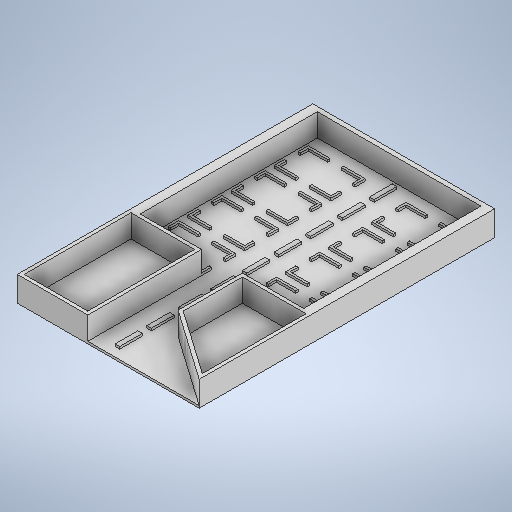
# Autodesk Inventor part: SchitaMacheta
Saved by Autodesk Inventor 2025 (Build 290162010, 162A)
## iProperties
Created: 2026-06-09
Part Number: SchitaMacheta
Material: Generic
Document SubType Name: Modeling
Designer: milot
Density: 1 g/cm^3
Appearance: Default
Author: milot
Autodesk Inventor part; units mm, degrees
ref_plane "YZ Plane" through (0, 0, 0) normal (1, 0, 0) x (0, 1, 0)
ref_plane "XZ Plane" through (0, 0, 0) normal (0, 1, 0) x (-1, 0, 0)
ref_plane "XY Plane" through (0, 0, 0) normal (0, 0, 1) x (1, 0, 0)
sketch "Sketch1" plane through (0, 0, 0) normal (0, 1, 0) x (-1, 0, 0)
  line L0 (-40, 65) -> (40, 65)
  line L1 (40, 65) -> (40, -65)
  line L2 (40, -65) -> (-40, -65)
  line L3 (-40, -65) -> (-40, 65)
  line L4 (-40, 65) -> (40, -65) construction
  line L5 (40, 65) -> (-40, -65) construction
  point P0 (0, 0)
  dimension "d0" = 130
  dimension "d1" = 80
  constraints: 12 end point, 2 midpoint, 2 parallel, 1 horizontal, 1 perpendicular
  measures "d0" distance of L0.end L1.end
  measures "d1" distance of L1.end L2.end
extrude "Extrusion1" add sketch "Sketch1" along normal blind 1
sketch "Sketch2" plane through (0, 1, 0) normal (0, 1, 0) x (1, 0, 0)
  line L0 (-40, -65) -> (40, -65) construction
  line L1 (0, -65) -> (-9, -65) construction
  line L2 (0, -65) -> (9, -65) construction
  line L3 (-9, -65) -> (9, -65)
  line L4 (9, -65) -> (9, 65)
  line L5 (-9, 85) -> (-9, -65)
  line L6 (1, -51) -> (-1, -51)
  line L7 (-1, -51) -> (-1, -61)
  line L8 (-1, -61) -> (1, -61)
  line L9 (1, -61) -> (1, -51)
  line L10 (1, -51) -> (-1, -61) construction
  line L11 (-1, -51) -> (1, -61) construction
  line L12 (-1, -61) -> (-1, -65) construction
  line L13 (1, -47) -> (1, -37)
  line L14 (1, -37) -> (-1, -37)
  line L15 (-1, -37) -> (-1, -47)
  line L16 (-1, -47) -> (1, -47)
  line L17 (1, -33) -> (1, -23)
  line L18 (1, -23) -> (-1, -23)
  line L19 (-1, -23) -> (-1, -33)
  line L20 (-1, -33) -> (1, -33)
  line L21 (1, -19) -> (1, -9)
  line L22 (1, -9) -> (-1, -9)
  line L23 (-1, -9) -> (-1, -19)
  line L24 (-1, -19) -> (1, -19)
  line L25 (1, -5) -> (1, 5)
  line L26 (1, 5) -> (-1, 5)
  line L27 (-1, 5) -> (-1, -5)
  line L28 (-1, -5) -> (1, -5)
  line L29 (1, 9) -> (1, 19)
  line L30 (1, 19) -> (-1, 19)
  line L31 (-1, 19) -> (-1, 9)
  line L32 (-1, 9) -> (1, 9)
  line L33 (1, 23) -> (1, 33)
  line L34 (1, 33) -> (-1, 33)
  line L35 (-1, 33) -> (-1, 23)
  line L36 (-1, 23) -> (1, 23)
  line L37 (1, 37) -> (1, 47)
  line L38 (1, 47) -> (-1, 47)
  line L39 (-1, 47) -> (-1, 37)
  line L40 (-1, 37) -> (1, 37)
  line L41 (1, 51) -> (1, 61)
  line L42 (1, 61) -> (-1, 61)
  line L43 (-1, 61) -> (-1, 51)
  line L44 (-1, 51) -> (1, 51)
  line L45 (1, 65) -> (1, 75)
  line L46 (1, 75) -> (-1, 75)
  line L47 (-1, 75) -> (-1, 65)
  line L48 (-1, 65) -> (1, 65)
  line L49 (-40, -65) -> (-9, -65)
  line L50 (-9, -65) -> (-9, -15)
  line L51 (-40, -15) -> (-40, -65)
  line L52 (40, -65) -> (9, -43.2936)
  line L53 (40, -65) -> (80.0993, -65) construction
  line L54 (40, -65) -> (40, -15)
  line L55 (40, -65) -> (40, 65) projected
  line L56 (40, -15) -> (9, -15)
  line L57 (24.5, -15) -> (24.5, -16.5) construction
  line L58 (9, -28) -> (10.5, -28) construction
  line L59 (40, -50) -> (38.5, -50) construction
  line L60 (20.0059, -51) -> (20.8663, -49.7713) construction
  line L61 (10.5, -28) -> (10.5, -16.5)
  line L62 (10.5, -16.5) -> (38.5, -16.5)
  line L63 (38.5, -16.5) -> (38.5, -62.1185)
  line L64 (38.5, -62.1185) -> (10.5, -42.5127)
  line L65 (10.5, -42.5127) -> (10.5, -28)
  line L66 (-40, -49.3093) -> (-38.5, -49.3093) construction
  line L67 (-24.5, -65) -> (-24.5, -63.5) construction
  line L68 (-38.5, -63.5) -> (-10.5, -63.5)
  line L69 (-10.5, -63.5) -> (-10.5, -16.5)
  line L70 (-10.5, -16.5) -> (-38.5, -16.5)
  line L71 (-38.5, -16.5) -> (-38.5, -63.5)
  line L72 (-38.5, -63.5) -> (-10.5, -63.5) construction
  line L73 (-40, 65) -> (-40, -65) construction
  line L74 (-40, 18) -> (-9, 18) construction
  line L75 (-34, -15) -> (-9, -15) construction
  line L76 (-34, -15) -> (-9, -15)
  line L77 (-24.5, -1) -> (-24.5, 0)
  line L78 (-18.5, -1) -> (-18.5, 0)
  line L79 (-18.5, -14) -> (-18.5, -15)
  line L80 (-24.5, -14) -> (-24.5, -15)
  line L81 (-10, -10.5) -> (-9, -10.5)
  line L82 (-10, -4.5) -> (-9, -4.5)
  line L83 (-33, -4.5) -> (-34, -4.5)
  line L84 (-33, -10.5) -> (-34, -10.5)
  line L85 (-10, -1) -> (-10, -4.5)
  line L86 (-10, -10.5) -> (-10, -14)
  line L87 (-9, -15) -> (-18.5, -15)
  line L88 (-21.5, -15) -> (-40, -15)
  line L89 (-10, -14) -> (-18.5, -14)
  line L90 (-24.5, -14) -> (-33, -14)
  line L91 (-33, -1) -> (-24.5, -1)
  line L92 (-18.5, -1) -> (-10, -1)
  line L93 (-33, -14) -> (-33, -10.5)
  line L94 (-33, -4.5) -> (-33, -1)
  line L95 (-34, 0) -> (-34, -4.5) construction
  line L96 (-34, -10.5) -> (-34, -15) construction
  line L97 (-34, 0) -> (-34, -4.5)
  line L98 (-34, -10.5) -> (-34, -15)
  line L99 (-9, 0) -> (-18.5, 0) construction
  line L100 (-24.5, 0) -> (-34, 0) construction
  line L101 (-9, 0) -> (-18.5, 0)
  line L102 (-24.5, 0) -> (-34, 0)
  line L103 (-9, -15) -> (-9, -10.5) construction
  line L104 (-9, -4.5) -> (-9, 0) construction
  line L105 (-9, -15) -> (-9, -10.5)
  line L106 (-9, -4.5) -> (-9, 0)
  line L107 (-33, 8.5) -> (-34, 8.5)
  line L108 (-34, 8.5) -> (-34, 4)
  line L109 (-33, 5) -> (-33, 8.5)
  line L110 (-24.5, 5) -> (-33, 5)
  line L111 (-24.5, 5) -> (-24.5, 4)
  line L112 (-18.5, 5) -> (-18.5, 4)
  line L113 (-10, 5) -> (-18.5, 5)
  line L114 (-10, 8.5) -> (-10, 5)
  line L115 (-10, 8.5) -> (-9, 8.5)
  line L116 (-10, 14.5) -> (-9, 14.5)
  line L117 (-10, 18) -> (-10, 14.5)
  line L118 (-18.5, 18) -> (-10, 18)
  line L119 (-9, 19) -> (-18.5, 19) construction
  line L120 (-18.5, 18) -> (-18.5, 19)
  line L121 (-24.5, 18) -> (-24.5, 19)
  line L122 (-9, 19) -> (-18.5, 19)
  line L123 (-33, 18) -> (-24.5, 18)
  line L124 (-33, 14.5) -> (-33, 18)
  line L125 (-33, 14.5) -> (-34, 14.5)
  line L126 (-34, 19) -> (-34, 14.5) construction
  line L127 (-34, 19) -> (-34, 14.5)
  line L128 (-24.5, 19) -> (-34, 19) construction
  line L129 (-24.5, 19) -> (-34, 19)
  line L130 (-33, 27.5) -> (-34, 27.5)
  line L131 (-34, 27.5) -> (-34, 23)
  line L132 (-33, 24) -> (-33, 27.5)
  line L133 (-24.5, 24) -> (-33, 24)
  line L134 (-24.5, 24) -> (-24.5, 23)
  line L135 (-18.5, 24) -> (-18.5, 23)
  line L136 (-10, 24) -> (-18.5, 24)
  line L137 (-10, 27.5) -> (-10, 24)
  line L138 (-10, 27.5) -> (-9, 27.5)
  line L139 (-10, 33.5) -> (-9, 33.5)
  line L140 (-10, 37) -> (-10, 33.5)
  line L141 (-18.5, 37) -> (-10, 37)
  line L142 (-9, 38) -> (-18.5, 38) construction
  line L143 (-18.5, 37) -> (-18.5, 38)
  line L144 (-24.5, 37) -> (-24.5, 38)
  line L145 (-9, 38) -> (-18.5, 38)
  line L146 (-33, 37) -> (-24.5, 37)
  line L147 (-33, 33.5) -> (-33, 37)
  line L148 (-33, 33.5) -> (-34, 33.5)
  line L149 (-34, 38) -> (-34, 33.5) construction
  line L150 (-34, 38) -> (-34, 33.5)
  line L151 (-24.5, 38) -> (-34, 38) construction
  line L152 (-24.5, 38) -> (-34, 38)
  line L153 (-33, 46.5) -> (-34, 46.5)
  line L154 (-34, 46.5) -> (-34, 42)
  line L155 (-33, 43) -> (-33, 46.5)
  line L156 (-24.5, 43) -> (-33, 43)
  line L157 (-24.5, 43) -> (-24.5, 42)
  line L158 (-18.5, 43) -> (-18.5, 42)
  line L159 (-10, 43) -> (-18.5, 43)
  line L160 (-10, 46.5) -> (-10, 43)
  line L161 (-10, 46.5) -> (-9, 46.5)
  line L162 (-10, 52.5) -> (-9, 52.5)
  line L163 (-10, 56) -> (-10, 52.5)
  line L164 (-18.5, 56) -> (-10, 56)
  line L165 (-9, 57) -> (-18.5, 57) construction
  line L166 (-18.5, 56) -> (-18.5, 57)
  line L167 (-24.5, 56) -> (-24.5, 57)
  line L168 (-9, 57) -> (-18.5, 57)
  line L169 (-33, 56) -> (-24.5, 56)
  line L170 (-33, 52.5) -> (-33, 56)
  line L171 (-33, 52.5) -> (-34, 52.5)
  line L172 (-34, 57) -> (-34, 52.5) construction
  line L173 (-34, 57) -> (-34, 52.5)
  line L174 (-24.5, 57) -> (-34, 57) construction
  line L175 (-24.5, 57) -> (-34, 57)
  line L176 (-34, 4) -> (-9, 4)
  line L177 (-34, 23) -> (-9, 23)
  line L178 (-34, 42) -> (-9, 42)
  line L179 (40, 65) -> (-40, 65) projected
  line L180 (0, 65) -> (0, -65)
  line L181 (40, 18) -> (9, 18) construction
  line L182 (24.5, -1) -> (24.5, 0)
  line L183 (18.5, -1) -> (18.5, 0)
  line L184 (18.5, -14) -> (18.5, -15)
  line L185 (24.5, -14) -> (24.5, -15)
  line L186 (10, -10.5) -> (9, -10.5)
  line L187 (10, -4.5) -> (9, -4.5)
  line L188 (33, -4.5) -> (34, -4.5)
  line L189 (33, -10.5) -> (34, -10.5)
  line L190 (10, -1) -> (10, -4.5)
  line L191 (10, -10.5) -> (10, -14)
  line L192 (10, -14) -> (18.5, -14)
  line L193 (24.5, -14) -> (33, -14)
  line L194 (33, -1) -> (24.5, -1)
  line L195 (18.5, -1) -> (10, -1)
  line L196 (33, -14) -> (33, -10.5)
  line L197 (33, -4.5) -> (33, -1)
  line L198 (34, 0) -> (34, -4.5) construction
  line L199 (34, -10.5) -> (34, -15) construction
  line L200 (34, 0) -> (34, -4.5)
  line L201 (34, -10.5) -> (34, -15)
  line L202 (9, 0) -> (18.5, 0) construction
  line L203 (24.5, 0) -> (34, 0) construction
  line L204 (9, 0) -> (18.5, 0)
  line L205 (24.5, 0) -> (34, 0)
  line L206 (33, 8.5) -> (34, 8.5)
  line L207 (34, 8.5) -> (34, 4)
  line L208 (33, 5) -> (33, 8.5)
  line L209 (24.5, 5) -> (33, 5)
  line L210 (24.5, 5) -> (24.5, 4)
  line L211 (18.5, 5) -> (18.5, 4)
  line L212 (10, 5) -> (18.5, 5)
  line L213 (10, 8.5) -> (10, 5)
  line L214 (10, 8.5) -> (9, 8.5)
  line L215 (10, 14.5) -> (9, 14.5)
  line L216 (10, 18) -> (10, 14.5)
  line L217 (18.5, 18) -> (10, 18)
  line L218 (9, 19) -> (18.5, 19) construction
  line L219 (18.5, 18) -> (18.5, 19)
  line L220 (24.5, 18) -> (24.5, 19)
  line L221 (9, 19) -> (18.5, 19)
  line L222 (33, 18) -> (24.5, 18)
  line L223 (33, 14.5) -> (33, 18)
  line L224 (33, 14.5) -> (34, 14.5)
  line L225 (34, 19) -> (34, 14.5) construction
  line L226 (34, 19) -> (34, 14.5)
  line L227 (24.5, 19) -> (34, 19) construction
  line L228 (24.5, 19) -> (34, 19)
  line L229 (33, 27.5) -> (34, 27.5)
  line L230 (34, 27.5) -> (34, 23)
  line L231 (33, 24) -> (33, 27.5)
  line L232 (24.5, 24) -> (33, 24)
  line L233 (24.5, 24) -> (24.5, 23)
  line L234 (18.5, 24) -> (18.5, 23)
  line L235 (10, 24) -> (18.5, 24)
  line L236 (10, 27.5) -> (10, 24)
  line L237 (10, 27.5) -> (9, 27.5)
  line L238 (10, 33.5) -> (9, 33.5)
  line L239 (10, 37) -> (10, 33.5)
  line L240 (18.5, 37) -> (10, 37)
  line L241 (9, 38) -> (18.5, 38) construction
  line L242 (18.5, 37) -> (18.5, 38)
  line L243 (24.5, 37) -> (24.5, 38)
  line L244 (9, 38) -> (18.5, 38)
  line L245 (33, 37) -> (24.5, 37)
  line L246 (33, 33.5) -> (33, 37)
  line L247 (33, 33.5) -> (34, 33.5)
  line L248 (34, 38) -> (34, 33.5) construction
  line L249 (34, 38) -> (34, 33.5)
  line L250 (24.5, 38) -> (34, 38) construction
  line L251 (24.5, 38) -> (34, 38)
  line L252 (33, 46.5) -> (34, 46.5)
  line L253 (34, 46.5) -> (34, 42)
  line L254 (33, 43) -> (33, 46.5)
  line L255 (24.5, 43) -> (33, 43)
  line L256 (24.5, 43) -> (24.5, 42)
  line L257 (18.5, 43) -> (18.5, 42)
  line L258 (10, 43) -> (18.5, 43)
  line L259 (10, 46.5) -> (10, 43)
  line L260 (10, 46.5) -> (9, 46.5)
  line L261 (10, 52.5) -> (9, 52.5)
  line L262 (10, 56) -> (10, 52.5)
  line L263 (18.5, 56) -> (10, 56)
  line L264 (9, 57) -> (18.5, 57) construction
  line L265 (18.5, 56) -> (18.5, 57)
  line L266 (24.5, 56) -> (24.5, 57)
  line L267 (9, 57) -> (18.5, 57)
  line L268 (33, 56) -> (24.5, 56)
  line L269 (33, 52.5) -> (33, 56)
  line L270 (33, 52.5) -> (34, 52.5)
  line L271 (34, 57) -> (34, 52.5) construction
  line L272 (34, 57) -> (34, 52.5)
  line L273 (24.5, 57) -> (34, 57) construction
  line L274 (24.5, 57) -> (34, 57)
  line L275 (34, 4) -> (9, 4)
  line L276 (34, 23) -> (9, 23)
  line L277 (34, 42) -> (9, 42)
  line L278 (-9, 65) -> (9, 65)
  line L279 (40, -15) -> (36, -15)
  line L280 (36, -15) -> (36, 65)
  line L281 (36, 65) -> (40, 65)
  line L282 (40, 65) -> (40, -15)
  line L283 (36, 65) -> (36, 63)
  line L284 (36, 63) -> (-36, 63)
  line L285 (-40, 63) -> (-40, 65)
  line L286 (-40, 65) -> (36, 65)
  line L287 (-40, 63) -> (-38.5, 63)
  line L288 (-36, 63) -> (-36, -15)
  line L289 (-36, -15) -> (-40, -15)
  line L290 (-40, -15) -> (-40, 63)
  point P0 (0, 0)
  point P1 (0, -56)
  dimension "d4" = 9
  dimension "d5" = 9
  dimension "d6" = 2
  dimension "d7" = 10
  dimension "d8" = 8
  dimension "d9" = 14
  dimension "d10" = 4
  dimension "d13" = 14
  dimension "d18" = 50
  dimension "d19" = 31
  dimension "d20" = 145
  dimension "d21" = 50
  dimension "d22" = 1.5
  dimension "d23" = 1.5
  dimension "d24" = 1.5
  dimension "d25" = 1.5
  dimension "d26" = 1.5
  dimension "d27" = 1.5
  dimension "d28" = 28
  dimension "d29" = 0
  dimension "d31" = 25
  dimension "d32" = 23
  dimension "d33" = 13
  dimension "d42" = 19
  dimension "d47" = 1.5
  dimension "d52" = 4
  dimension "d53" = 2
  dimension "d54" = 4
  constraints: 570 end point, 108 vertical alignment, 101 symmetric about line, 88 parallel, 54 collinear, 26 perpendicular, 14 horizontal, 14 point on line, 6 midpoint, 5 vertical, 19 other
  measures "d4" distance of L1.start L1.end
  measures "d5" distance of L1.start L2.end
  measures "d6" distance of L8.end L7.end
  measures "d7" distance of L7.end L6.end
  measures "d9" distance between parallel lines of L0 L6
  measures "d10" distance of L7.end L12.end
  measures "d13" distance of L8.end L13.start
  measures "d18" distance of L50.end L1.end
  measures "d19" distance of L0.start L1.end
  measures "d20" angle of L53 L52
  measures "d21" distance of L0.end L54.end
  measures "d22" distance of L57.start L57.end
  measures "d23" distance of L58.start L58.end
  measures "d24" distance of L59.start L59.end
  measures "d25" distance of L60.start L60.end
  measures "d26" distance of L66.start L66.end
  measures "d27" distance of L67.start L67.end
  measures "d28" distance of L68.start L68.end
  measures "d29" distance between parallel lines of L68 L72
  measures "d31" distance of L95.start L99.start
  measures "d32" distance of L91.start L85.start
  measures "d33" distance of L90.end L91.start
  measures "d42" distance of L84.start L107.start
  measures "d47" distance between parallel lines of L76 L70
  measures "d52" distance of L54.end L279.end
  measures "d53" distance of L280.end L283.end
  measures "d54" distance of L284.end L285.start
extrude "Extrusion2" add sketch "Sketch2" along normal blind 10 contours L49 L51 L88 L76 L5 | L290 L285 L179 L5 L284 L288 L88 | L4 L56 L54 L52 | L56 L280 L179 L55 | L5 L179 L48 L180 L284 | L180 L48 L179 L4 L284 | L280 L284 L4 L179
extrude "Extrusion3" add sketch "Sketch2" along normal blind 1 contours L76 L79 L89 L86 L81 L5 | L180 L6 L9 L8 | L8 L7 L6 L180 | L176 L108 L107 L109 L110 L111 | L177 L131 L130 L132 L133 L134 | L178 L154 L153 L155 L156 L157 | L82 L85 L92 L78 L101 L5 | L4 L186 L191 L192 L184 L56 | L180 L14 L13 L16 | L16 L15 L14 L180 | L76 L98 L84 L93 L90 L80 | L256 L255 L254 L252 L253 L277 | L233 L232 L231 L229 L230 L276 | L210 L209 L208 L206 L207 L275 | L176 L112 L113 L114 L115 L5 | L4 L204 L183 L195 L190 L187 | L185 L193 L196 L189 L201 L56 | L180 L18 L17 L20 | L20 L19 L18 L180 | L5 L162 L163 L164 L166 L168 | L116 L117 L118 L120 L122 L5 | L180 L44 L43 L42 | L42 L41 L44 L180 | L4 L214 L213 L212 L211 L275 | L180 L22 L21 L24 | L24 L23 L22 L180 | L5 L178 L158 L159 L160 L161 | L267 L265 L263 L262 L261 L4 | L177 L135 L136 L137 L138 L5 | L180 L40 L39 L38 | L38 L37 L40 L180 | L4 L221 L219 L217 L216 L215 | L180 L26 L25 L28 | L28 L27 L26 L180 | L5 L139 L140 L141 L143 L145 | L260 L259 L258 L257 L277 L4 | L180 L36 L35 L34 | L34 L33 L36 L180 | L4 L237 L236 L235 L234 L276 | L180 L30 L29 L32 | L32 L31 L30 L180 | L244 L242 L240 L239 L238 L4 | L91 L94 L83 L97 L102 L77 | L123 L124 L125 L127 L129 L121 | L146 L147 L148 L150 L152 L144 | L169 L170 L171 L173 L175 L167 | L182 L205 L200 L188 L197 L194 | L220 L228 L226 L224 L223 L222 | L243 L251 L249 L247 L246 L245 | L266 L274 L272 L270 L269 L268
body "Solid1"
